Autodesk Fusion 360 part; units mm, degrees
(part 2 of 2)
sketch "Back Honeycomb" plane through (0, 0, 0) normal (0, 0, -1) x (-1, 0, 0)
  line L0 (-88.9, 0) -> (0, 0)
  line L1 (0, 0) -> (0, 22)
  line L2 (0, 22) -> (-88.9, 22)
  line L3 (-88.9, 22) -> (-88.9, 0)
  line L4 (-41.45, 11) -> (-42.95, 13.5981)
  line L5 (-42.95, 13.5981) -> (-45.95, 13.5981)
  line L6 (-45.95, 13.5981) -> (-47.45, 11)
  line L7 (-47.45, 11) -> (-45.95, 8.4019)
  line L8 (-45.95, 8.4019) -> (-42.95, 8.4019)
  line L9 (-42.95, 8.4019) -> (-41.45, 11)
  line L10 (-35.45, 11) -> (-33.95, 8.4019)
  line L11 (-33.95, 8.4019) -> (-30.95, 8.4019)
  line L12 (-30.95, 8.4019) -> (-29.45, 11)
  line L13 (-29.45, 11) -> (-30.95, 13.5981)
  line L14 (-30.95, 13.5981) -> (-33.95, 13.5981)
  line L15 (-33.95, 13.5981) -> (-35.45, 11)
  line L16 (-86.9, 20) -> (-2, 20)
  line L17 (-2, 20) -> (-2, 2)
  line L18 (-2, 2) -> (-86.9, 2)
  line L19 (-86.9, 2) -> (-86.9, 20)
  line L20 (-23.45, 11) -> (-21.95, 8.4019)
  line L21 (-21.95, 8.4019) -> (-18.95, 8.4019)
  line L22 (-18.95, 8.4019) -> (-17.45, 11)
  line L23 (-17.45, 11) -> (-18.95, 13.5981)
  line L24 (-18.95, 13.5981) -> (-21.95, 13.5981)
  line L25 (-21.95, 13.5981) -> (-23.45, 11)
  line L26 (-11.45, 11) -> (-9.95, 8.4019)
  line L27 (-9.95, 8.4019) -> (-6.95, 8.4019)
  line L28 (-6.95, 8.4019) -> (-5.45, 11)
  line L29 (-5.45, 11) -> (-6.95, 13.5981)
  line L30 (-6.95, 13.5981) -> (-9.95, 13.5981)
  line L31 (-9.95, 13.5981) -> (-11.45, 11)
  line L32 (-59.45, 11) -> (-57.95, 8.4019)
  line L33 (-57.95, 8.4019) -> (-54.95, 8.4019)
  line L34 (-54.95, 8.4019) -> (-53.45, 11)
  line L35 (-53.45, 11) -> (-54.95, 13.5981)
  line L36 (-54.95, 13.5981) -> (-57.95, 13.5981)
  line L37 (-57.95, 13.5981) -> (-59.45, 11)
  line L38 (-71.45, 11) -> (-69.95, 8.4019)
  line L39 (-69.95, 8.4019) -> (-66.95, 8.4019)
  line L40 (-66.95, 8.4019) -> (-65.45, 11)
  line L41 (-65.45, 11) -> (-66.95, 13.5981)
  line L42 (-66.95, 13.5981) -> (-69.95, 13.5981)
  line L43 (-69.95, 13.5981) -> (-71.45, 11)
  line L44 (-83.45, 11) -> (-81.95, 8.4019)
  line L45 (-81.95, 8.4019) -> (-78.95, 8.4019)
  line L46 (-78.95, 8.4019) -> (-77.45, 11)
  line L47 (-77.45, 11) -> (-78.95, 13.5981)
  line L48 (-78.95, 13.5981) -> (-81.95, 13.5981)
  line L49 (-81.95, 13.5981) -> (-83.45, 11)
  line L50 (-77.45, 14.5) -> (-75.95, 11.9019)
  line L51 (-75.95, 11.9019) -> (-72.95, 11.9019)
  line L52 (-72.95, 11.9019) -> (-71.45, 14.5)
  line L53 (-71.45, 14.5) -> (-72.95, 17.0981)
  line L54 (-72.95, 17.0981) -> (-75.95, 17.0981)
  line L55 (-75.95, 17.0981) -> (-77.45, 14.5)
  line L56 (-65.45, 14.5) -> (-63.95, 11.9019)
  line L57 (-63.95, 11.9019) -> (-60.95, 11.9019)
  line L58 (-60.95, 11.9019) -> (-59.45, 14.5)
  line L59 (-59.45, 14.5) -> (-60.95, 17.0981)
  line L60 (-60.95, 17.0981) -> (-63.95, 17.0981)
  line L61 (-63.95, 17.0981) -> (-65.45, 14.5)
  line L62 (-53.45, 14.5) -> (-51.95, 11.9019)
  line L63 (-51.95, 11.9019) -> (-48.95, 11.9019)
  line L64 (-48.95, 11.9019) -> (-47.45, 14.5)
  line L65 (-47.45, 14.5) -> (-48.95, 17.0981)
  line L66 (-48.95, 17.0981) -> (-51.95, 17.0981)
  line L67 (-51.95, 17.0981) -> (-53.45, 14.5)
  line L68 (-41.45, 14.5) -> (-39.95, 11.9019)
  line L69 (-39.95, 11.9019) -> (-36.95, 11.9019)
  line L70 (-36.95, 11.9019) -> (-35.45, 14.5)
  line L71 (-35.45, 14.5) -> (-36.95, 17.0981)
  line L72 (-36.95, 17.0981) -> (-39.95, 17.0981)
  line L73 (-39.95, 17.0981) -> (-41.45, 14.5)
  line L74 (-29.45, 14.5) -> (-27.95, 11.9019)
  line L75 (-27.95, 11.9019) -> (-24.95, 11.9019)
  line L76 (-24.95, 11.9019) -> (-23.45, 14.5)
  line L77 (-23.45, 14.5) -> (-24.95, 17.0981)
  line L78 (-24.95, 17.0981) -> (-27.95, 17.0981)
  line L79 (-27.95, 17.0981) -> (-29.45, 14.5)
  line L80 (-17.45, 14.5) -> (-15.95, 11.9019)
  line L81 (-15.95, 11.9019) -> (-12.95, 11.9019)
  line L82 (-12.95, 11.9019) -> (-11.45, 14.5)
  line L83 (-11.45, 14.5) -> (-12.95, 17.0981)
  line L84 (-12.95, 17.0981) -> (-15.95, 17.0981)
  line L85 (-15.95, 17.0981) -> (-17.45, 14.5)
  line L86 (-71.45, 7.5) -> (-72.95, 10.0981)
  line L87 (-72.95, 10.0981) -> (-75.95, 10.0981)
  line L88 (-75.95, 10.0981) -> (-77.45, 7.5)
  line L89 (-77.45, 7.5) -> (-75.95, 4.9019)
  line L90 (-75.95, 4.9019) -> (-72.95, 4.9019)
  line L91 (-72.95, 4.9019) -> (-71.45, 7.5)
  line L92 (-59.45, 7.5) -> (-60.95, 10.0981)
  line L93 (-60.95, 10.0981) -> (-63.95, 10.0981)
  line L94 (-63.95, 10.0981) -> (-65.45, 7.5)
  line L95 (-65.45, 7.5) -> (-63.95, 4.9019)
  line L96 (-60.95, 4.9019) -> (-59.45, 7.5)
  line L97 (-63.95, 4.9019) -> (-60.95, 4.9019)
  line L98 (-47.45, 7.5) -> (-48.95, 10.0981)
  line L99 (-48.95, 10.0981) -> (-51.95, 10.0981)
  line L100 (-51.95, 10.0981) -> (-53.45, 7.5)
  line L101 (-53.45, 7.5) -> (-51.95, 4.9019)
  line L102 (-48.95, 4.9019) -> (-47.45, 7.5)
  line L103 (-51.95, 4.9019) -> (-48.95, 4.9019)
  line L104 (-35.45, 7.5) -> (-36.95, 10.0981)
  line L105 (-36.95, 10.0981) -> (-39.95, 10.0981)
  line L106 (-39.95, 10.0981) -> (-41.45, 7.5)
  line L107 (-41.45, 7.5) -> (-39.95, 4.9019)
  line L108 (-36.95, 4.9019) -> (-35.45, 7.5)
  line L109 (-39.95, 4.9019) -> (-36.95, 4.9019)
  line L110 (-23.45, 7.5) -> (-24.95, 10.0981)
  line L111 (-24.95, 10.0981) -> (-27.95, 10.0981)
  line L112 (-27.95, 10.0981) -> (-29.45, 7.5)
  line L113 (-29.45, 7.5) -> (-27.95, 4.9019)
  line L114 (-24.95, 4.9019) -> (-23.45, 7.5)
  line L115 (-27.95, 4.9019) -> (-24.95, 4.9019)
  line L116 (-11.45, 7.5) -> (-12.95, 10.0981)
  line L117 (-12.95, 10.0981) -> (-15.95, 10.0981)
  line L118 (-15.95, 10.0981) -> (-17.45, 7.5)
  line L119 (-17.45, 7.5) -> (-15.95, 4.9019)
  line L120 (-12.95, 4.9019) -> (-11.45, 7.5)
  line L121 (-15.95, 4.9019) -> (-12.95, 4.9019)
  line L122 (-83.45, 18) -> (-81.95, 15.4019)
  line L123 (-81.95, 15.4019) -> (-78.95, 15.4019)
  line L124 (-78.95, 15.4019) -> (-77.45, 18)
  line L125 (-77.45, 18) -> (-78.95, 20.5981)
  line L126 (-78.95, 20.5981) -> (-81.95, 20.5981)
  line L127 (-81.95, 20.5981) -> (-83.45, 18)
  line L128 (-71.45, 18) -> (-69.95, 15.4019)
  line L129 (-69.95, 15.4019) -> (-66.95, 15.4019)
  line L130 (-66.95, 15.4019) -> (-65.45, 18)
  line L131 (-65.45, 18) -> (-66.95, 20.5981)
  line L132 (-69.95, 20.5981) -> (-71.45, 18)
  line L133 (-66.95, 20.5981) -> (-69.95, 20.5981)
  line L134 (-59.45, 18) -> (-57.95, 15.4019)
  line L135 (-57.95, 15.4019) -> (-54.95, 15.4019)
  line L136 (-54.95, 15.4019) -> (-53.45, 18)
  line L137 (-53.45, 18) -> (-54.95, 20.5981)
  line L138 (-57.95, 20.5981) -> (-59.45, 18)
  line L139 (-54.95, 20.5981) -> (-57.95, 20.5981)
  line L140 (-47.45, 18) -> (-45.95, 15.4019)
  line L141 (-45.95, 15.4019) -> (-42.95, 15.4019)
  line L142 (-42.95, 15.4019) -> (-41.45, 18)
  line L143 (-41.45, 18) -> (-42.95, 20.5981)
  line L144 (-45.95, 20.5981) -> (-47.45, 18)
  line L145 (-42.95, 20.5981) -> (-45.95, 20.5981)
  line L146 (-35.45, 18) -> (-33.95, 15.4019)
  line L147 (-33.95, 15.4019) -> (-30.95, 15.4019)
  line L148 (-30.95, 15.4019) -> (-29.45, 18)
  line L149 (-29.45, 18) -> (-30.95, 20.5981)
  line L150 (-33.95, 20.5981) -> (-35.45, 18)
  line L151 (-30.95, 20.5981) -> (-33.95, 20.5981)
  line L152 (-23.45, 18) -> (-21.95, 15.4019)
  line L153 (-21.95, 15.4019) -> (-18.95, 15.4019)
  line L154 (-18.95, 15.4019) -> (-17.45, 18)
  line L155 (-17.45, 18) -> (-18.95, 20.5981)
  line L156 (-21.95, 20.5981) -> (-23.45, 18)
  line L157 (-18.95, 20.5981) -> (-21.95, 20.5981)
  line L158 (-11.45, 18) -> (-9.95, 15.4019)
  line L159 (-9.95, 15.4019) -> (-6.95, 15.4019)
  line L160 (-6.95, 15.4019) -> (-5.45, 18)
  line L161 (-5.45, 18) -> (-6.95, 20.5981)
  line L162 (-9.95, 20.5981) -> (-11.45, 18)
  line L163 (-6.95, 20.5981) -> (-9.95, 20.5981)
  line L164 (-83.45, 4) -> (-81.95, 1.4019)
  line L165 (-81.95, 1.4019) -> (-78.95, 1.4019)
  line L166 (-78.95, 1.4019) -> (-77.45, 4)
  line L167 (-77.45, 4) -> (-78.95, 6.5981)
  line L168 (-78.95, 6.5981) -> (-81.95, 6.5981)
  line L169 (-81.95, 6.5981) -> (-83.45, 4)
  line L170 (-71.45, 4) -> (-69.95, 1.4019)
  line L171 (-69.95, 1.4019) -> (-66.95, 1.4019)
  line L172 (-66.95, 1.4019) -> (-65.45, 4)
  line L173 (-65.45, 4) -> (-66.95, 6.5981)
  line L174 (-69.95, 6.5981) -> (-71.45, 4)
  line L175 (-66.95, 6.5981) -> (-69.95, 6.5981)
  line L176 (-59.45, 4) -> (-57.95, 1.4019)
  line L177 (-57.95, 1.4019) -> (-54.95, 1.4019)
  line L178 (-54.95, 1.4019) -> (-53.45, 4)
  line L179 (-53.45, 4) -> (-54.95, 6.5981)
  line L180 (-57.95, 6.5981) -> (-59.45, 4)
  line L181 (-54.95, 6.5981) -> (-57.95, 6.5981)
  line L182 (-47.45, 4) -> (-45.95, 1.4019)
  line L183 (-45.95, 1.4019) -> (-42.95, 1.4019)
  line L184 (-42.95, 1.4019) -> (-41.45, 4)
  line L185 (-41.45, 4) -> (-42.95, 6.5981)
  line L186 (-45.95, 6.5981) -> (-47.45, 4)
  line L187 (-42.95, 6.5981) -> (-45.95, 6.5981)
  line L188 (-35.45, 4) -> (-33.95, 1.4019)
  line L189 (-33.95, 1.4019) -> (-30.95, 1.4019)
  line L190 (-30.95, 1.4019) -> (-29.45, 4)
  line L191 (-29.45, 4) -> (-30.95, 6.5981)
  line L192 (-33.95, 6.5981) -> (-35.45, 4)
  line L193 (-30.95, 6.5981) -> (-33.95, 6.5981)
  line L194 (-23.45, 4) -> (-21.95, 1.4019)
  line L195 (-21.95, 1.4019) -> (-18.95, 1.4019)
  line L196 (-18.95, 1.4019) -> (-17.45, 4)
  line L197 (-17.45, 4) -> (-18.95, 6.5981)
  line L198 (-21.95, 6.5981) -> (-23.45, 4)
  line L199 (-18.95, 6.5981) -> (-21.95, 6.5981)
  line L200 (-11.45, 4) -> (-9.95, 1.4019)
  line L201 (-9.95, 1.4019) -> (-6.95, 1.4019)
  line L202 (-6.95, 1.4019) -> (-5.45, 4)
  line L203 (-5.45, 4) -> (-6.95, 6.5981)
  line L204 (-9.95, 6.5981) -> (-11.45, 4)
  line L205 (-6.95, 6.5981) -> (-9.95, 6.5981)
  line L206 (0.55, 14.5) -> (-0.95, 17.0981)
  line L207 (-0.95, 17.0981) -> (-3.95, 17.0981)
  line L208 (-3.95, 17.0981) -> (-5.45, 14.5)
  line L209 (-5.45, 14.5) -> (-3.95, 11.9019)
  line L210 (-3.95, 11.9019) -> (-0.95, 11.9019)
  line L211 (-0.95, 11.9019) -> (0.55, 14.5)
  line L212 (-5.45, 7.5) -> (-3.95, 4.9019)
  line L213 (-3.95, 4.9019) -> (-0.95, 4.9019)
  line L214 (-0.95, 4.9019) -> (0.55, 7.5)
  line L215 (0.55, 7.5) -> (-0.95, 10.0981)
  line L216 (-3.95, 10.0981) -> (-5.45, 7.5)
  line L217 (-0.95, 10.0981) -> (-3.95, 10.0981)
  line L218 (-89.45, 14.5) -> (-87.95, 11.9019)
  line L219 (-87.95, 11.9019) -> (-84.95, 11.9019)
  line L220 (-84.95, 11.9019) -> (-83.45, 14.5)
  line L221 (-83.45, 14.5) -> (-84.95, 17.0981)
  line L222 (-84.95, 17.0981) -> (-87.95, 17.0981)
  line L223 (-87.95, 17.0981) -> (-89.45, 14.5)
  line L224 (-89.45, 7.5) -> (-87.95, 4.9019)
  line L225 (-87.95, 4.9019) -> (-84.95, 4.9019)
  line L226 (-84.95, 4.9019) -> (-83.45, 7.5)
  line L227 (-83.45, 7.5) -> (-84.95, 10.0981)
  line L228 (-87.95, 10.0981) -> (-89.45, 7.5)
  line L229 (-84.95, 10.0981) -> (-87.95, 10.0981)
  line L230 (-77.45, 21.5) -> (-75.95, 18.9019)
  line L231 (-75.95, 18.9019) -> (-72.95, 18.9019)
  line L232 (-72.95, 18.9019) -> (-71.45, 21.5)
  line L233 (-71.45, 21.5) -> (-72.95, 24.0981)
  line L234 (-72.95, 24.0981) -> (-75.95, 24.0981)
  line L235 (-75.95, 24.0981) -> (-77.45, 21.5)
  line L236 (-65.45, 21.5) -> (-63.95, 18.9019)
  line L237 (-63.95, 18.9019) -> (-60.95, 18.9019)
  line L238 (-60.95, 18.9019) -> (-59.45, 21.5)
  line L239 (-59.45, 21.5) -> (-60.95, 24.0981)
  line L240 (-63.95, 24.0981) -> (-65.45, 21.5)
  line L241 (-60.95, 24.0981) -> (-63.95, 24.0981)
  line L242 (-53.45, 21.5) -> (-51.95, 18.9019)
  line L243 (-51.95, 18.9019) -> (-48.95, 18.9019)
  line L244 (-48.95, 18.9019) -> (-47.45, 21.5)
  line L245 (-47.45, 21.5) -> (-48.95, 24.0981)
  line L246 (-51.95, 24.0981) -> (-53.45, 21.5)
  line L247 (-48.95, 24.0981) -> (-51.95, 24.0981)
  line L248 (-41.45, 21.5) -> (-39.95, 18.9019)
  line L249 (-39.95, 18.9019) -> (-36.95, 18.9019)
  line L250 (-36.95, 18.9019) -> (-35.45, 21.5)
  line L251 (-35.45, 21.5) -> (-36.95, 24.0981)
  line L252 (-39.95, 24.0981) -> (-41.45, 21.5)
  line L253 (-36.95, 24.0981) -> (-39.95, 24.0981)
  line L254 (-29.45, 21.5) -> (-27.95, 18.9019)
  line L255 (-27.95, 18.9019) -> (-24.95, 18.9019)
  line L256 (-24.95, 18.9019) -> (-23.45, 21.5)
  line L257 (-23.45, 21.5) -> (-24.95, 24.0981)
  line L258 (-27.95, 24.0981) -> (-29.45, 21.5)
  line L259 (-24.95, 24.0981) -> (-27.95, 24.0981)
  line L260 (-17.45, 21.5) -> (-15.95, 18.9019)
  line L261 (-15.95, 18.9019) -> (-12.95, 18.9019)
  line L262 (-12.95, 18.9019) -> (-11.45, 21.5)
  line L263 (-11.45, 21.5) -> (-12.95, 24.0981)
  line L264 (-15.95, 24.0981) -> (-17.45, 21.5)
  line L265 (-12.95, 24.0981) -> (-15.95, 24.0981)
  line L266 (-5.45, 21.5) -> (-3.95, 18.9019)
  line L267 (-3.95, 18.9019) -> (-0.95, 18.9019)
  line L268 (-0.95, 18.9019) -> (0.55, 21.5)
  line L269 (0.55, 21.5) -> (-0.95, 24.0981)
  line L270 (-3.95, 24.0981) -> (-5.45, 21.5)
  line L271 (-0.95, 24.0981) -> (-3.95, 24.0981)
  line L272 (-77.45, 0.5) -> (-75.95, -2.0981)
  line L273 (-75.95, -2.0981) -> (-72.95, -2.0981)
  line L274 (-72.95, -2.0981) -> (-71.45, 0.5)
  line L275 (-71.45, 0.5) -> (-72.95, 3.0981)
  line L276 (-72.95, 3.0981) -> (-75.95, 3.0981)
  line L277 (-75.95, 3.0981) -> (-77.45, 0.5)
  line L278 (-65.45, 0.5) -> (-63.95, -2.0981)
  line L279 (-63.95, -2.0981) -> (-60.95, -2.0981)
  line L280 (-60.95, -2.0981) -> (-59.45, 0.5)
  line L281 (-59.45, 0.5) -> (-60.95, 3.0981)
  line L282 (-63.95, 3.0981) -> (-65.45, 0.5)
  line L283 (-60.95, 3.0981) -> (-63.95, 3.0981)
  line L284 (-53.45, 0.5) -> (-51.95, -2.0981)
  line L285 (-51.95, -2.0981) -> (-48.95, -2.0981)
  line L286 (-48.95, -2.0981) -> (-47.45, 0.5)
  line L287 (-47.45, 0.5) -> (-48.95, 3.0981)
  line L288 (-51.95, 3.0981) -> (-53.45, 0.5)
  line L289 (-48.95, 3.0981) -> (-51.95, 3.0981)
  line L290 (-41.45, 0.5) -> (-39.95, -2.0981)
  line L291 (-39.95, -2.0981) -> (-36.95, -2.0981)
  line L292 (-36.95, -2.0981) -> (-35.45, 0.5)
  line L293 (-35.45, 0.5) -> (-36.95, 3.0981)
  line L294 (-39.95, 3.0981) -> (-41.45, 0.5)
  line L295 (-36.95, 3.0981) -> (-39.95, 3.0981)
  line L296 (-29.45, 0.5) -> (-27.95, -2.0981)
  line L297 (-27.95, -2.0981) -> (-24.95, -2.0981)
  line L298 (-24.95, -2.0981) -> (-23.45, 0.5)
  line L299 (-23.45, 0.5) -> (-24.95, 3.0981)
  line L300 (-27.95, 3.0981) -> (-29.45, 0.5)
  line L301 (-24.95, 3.0981) -> (-27.95, 3.0981)
  line L302 (-17.45, 0.5) -> (-15.95, -2.0981)
  line L303 (-15.95, -2.0981) -> (-12.95, -2.0981)
  line L304 (-12.95, -2.0981) -> (-11.45, 0.5)
  line L305 (-11.45, 0.5) -> (-12.95, 3.0981)
  line L306 (-15.95, 3.0981) -> (-17.45, 0.5)
  line L307 (-12.95, 3.0981) -> (-15.95, 3.0981)
  line L308 (-5.45, 0.5) -> (-3.95, -2.0981)
  line L309 (-3.95, -2.0981) -> (-0.95, -2.0981)
  line L310 (-0.95, -2.0981) -> (0.55, 0.5)
  line L311 (0.55, 0.5) -> (-0.95, 3.0981)
  line L312 (-3.95, 3.0981) -> (-5.45, 0.5)
  line L313 (-0.95, 3.0981) -> (-3.95, 3.0981)
  line L314 (-89.45, 21.5) -> (-87.95, 18.9019)
  line L315 (-87.95, 18.9019) -> (-84.95, 18.9019)
  line L316 (-84.95, 18.9019) -> (-83.45, 21.5)
  line L317 (-83.45, 21.5) -> (-84.95, 24.0981)
  line L318 (-84.95, 24.0981) -> (-87.95, 24.0981)
  line L319 (-87.95, 24.0981) -> (-89.45, 21.5)
  line L320 (-83.45, 0.5) -> (-84.95, 3.0981)
  line L321 (-84.95, 3.0981) -> (-87.95, 3.0981)
  line L322 (-87.95, 3.0981) -> (-89.45, 0.5)
  line L323 (-89.45, 0.5) -> (-87.95, -2.0981)
  line L324 (-87.95, -2.0981) -> (-84.95, -2.0981)
  line L325 (-84.95, -2.0981) -> (-83.45, 0.5)
  line L326 (-8.45, 20.5981) -> (-8.45, 15.4019) construction
  line L327 (-32.45, 20.5981) -> (-32.45, 15.4019) construction
  line L328 (-44.45, 20.5981) -> (-44.45, 15.4019) construction
  line L329 (-80.45, 20.5981) -> (-80.45, 15.4019) construction
  line L330 (-88.9, 18.0734) -> (0, 18) construction
  point P0 (-44.45, 11)
  point P1 (-44.45, 11)
  point P2 (-44.45, 11)
  point P3 (-2, 2)
  dimension "d240" = 5.1962
  dimension "d241" = 5.45
  dimension "d242" = 88.9
  measures "d240" distance of L326.start L326.end
  measures "d241" distance of L160.end L330.end
  measures "d242" distance of L330.end L330.start
extrude "Extrude11" cut sketch "Back Honeycomb" against normal blind 2 contours L18 L19 L320 L321 | L18 L275 L276 L277 | L18 L164 L166 L167 L168 L169 | L19 L225 L226 L227 L229 | L18 L281 L282 L283 | L18 L170 L172 L173 L174 L175 | L19 L219 L220 L221 L222 | L18 L287 L288 L289 | L18 L176 L178 L179 L180 L181 | L16 L19 L315 L316 | L18 L293 L294 L295 | L18 L182 L184 L185 L186 L187 | L16 L230 L231 L232 | L16 L122 L123 L124 L125 L127 | L18 L299 L300 L301 | L18 L188 L190 L191 L192 L193 | L16 L236 L237 L238 | L16 L128 L129 L130 L131 L132 | L18 L305 L306 L307 | L18 L194 L196 L197 L198 L199 | L16 L242 L243 L244 | L16 L134 L135 L136 L137 L138 | L17 L18 L312 L313 | L18 L200 L202 L203 L204 L205 | L16 L248 L249 L250 | L16 L140 L141 L142 L143 L144 | L17 L212 L213 L216 L217 | L16 L254 L255 L256 | L16 L146 L147 L148 L149 L150 | L17 L207 L208 L209 L210 | L16 L260 L261 L262 | L16 L152 L153 L154 L155 L156 | L16 L17 L266 L267 | L16 L158 L159 L160 L161 L162 | L4 L5 L6 L7 L8 L9 | L10 L11 L12 L13 L14 L15 | L20 L21 L22 L23 L24 L25 | L26 L27 L28 L29 L30 L31 | L32 L33 L34 L35 L36 L37 | L38 L39 L40 L41 L42 L43 | L44 L45 L46 L47 L48 L49 | L50 L51 L52 L53 L54 L55 | L56 L57 L58 L59 L60 L61 | L62 L63 L64 L65 L66 L67 | L68 L69 L70 L71 L72 L73 | L74 L75 L76 L77 L78 L79 | L80 L81 L82 L83 L84 L85 | L86 L87 L88 L89 L90 L91 | L92 L93 L94 L95 L96 L97 | L98 L99 L100 L101 L102 L103 | L104 L105 L106 L107 L108 L109 | L110 L111 L112 L113 L114 L115 | L116 L117 L118 L119 L120 L121 bodies 2
extrude "Extrude12" cut sketch "Bottom Honeycomb" along normal blind 2 contours L493 L513 L514 L515 L517 | L485 L486 L487 L492 A2 | L493 L507 L508 L509 L511 | L492 L493 A2 L556 | L493 L500 L501 L504 L505 | L422 L423 L424 L425 L427 L492 | L476 L477 L478 L492 | L428 L429 L430 L431 A1 | L392 L393 L394 L395 L396 L492 | L470 L471 L472 L492 | L362 L363 L364 L365 L367 L490 | L386 L387 L388 L389 L390 L490 | L398 L399 L400 L401 L402 L492 | L368 L369 L372 L490 A8 | L491 L524 L529 | L442 L443 L444 L445 A0 | L380 L381 L382 L383 L384 L490 | L369 L370 L371 L490 A8 | L464 L465 L466 L492 | L491 L530 L534 | L374 L375 L376 L377 L378 L490 | L404 L405 L406 L407 L408 L492 | L491 L536 L540 | L458 L459 L460 L492 | L446 L449 L450 L451 A3 | L410 L411 L412 L413 L414 L492 | L491 A3 L542 | L452 L453 L454 L492 | L492 A3 L497 L498 L499 | L416 L417 L418 L419 L420 L492 bodies 1
sketch "Non-USB Honeycomb" plane through (88.9, 0, 0) normal (1, 0, 0) x (0, 0, -1)
  line L0 (-47.6, 0) -> (0, 0)
  line L1 (0, 0) -> (0, 22)
  line L2 (0, 22) -> (-47.6, 22)
  line L3 (-47.6, 22) -> (-47.6, 0)
  line L4 (-45.6, 20) -> (-2, 20)
  line L5 (-2, 20) -> (-2, 2)
  line L6 (-2, 2) -> (-45.6, 2)
  line L7 (-45.6, 2) -> (-45.6, 20)
  line L8 (-45.6, 11) -> (-2, 11) construction
  line L9 (-23.8, 20) -> (-23.8, 2) construction
  line L10 (-20.8, 11) -> (-22.3, 13.5981)
  line L11 (-22.3, 13.5981) -> (-25.3, 13.5981)
  line L12 (-25.3, 13.5981) -> (-26.8, 11)
  line L13 (-26.8, 11) -> (-25.3, 8.4019)
  line L14 (-25.3, 8.4019) -> (-22.3, 8.4019)
  line L15 (-22.3, 8.4019) -> (-20.8, 11)
  line L16 (-14.8, 11) -> (-13.3, 8.4019)
  line L17 (-13.3, 8.4019) -> (-10.3, 8.4019)
  line L18 (-10.3, 8.4019) -> (-8.8, 11)
  line L19 (-8.8, 11) -> (-10.3, 13.5981)
  line L20 (-10.3, 13.5981) -> (-13.3, 13.5981)
  line L21 (-13.3, 13.5981) -> (-14.8, 11)
  line L22 (-2.8, 11) -> (-1.3, 8.4019)
  line L23 (-1.3, 8.4019) -> (1.7, 8.4019)
  line L24 (1.7, 8.4019) -> (3.2, 11)
  line L25 (3.2, 11) -> (1.7, 13.5981)
  line L26 (1.7, 13.5981) -> (-1.3, 13.5981)
  line L27 (-1.3, 13.5981) -> (-2.8, 11)
  line L28 (-38.8, 11) -> (-37.3, 8.4019)
  line L29 (-37.3, 8.4019) -> (-34.3, 8.4019)
  line L30 (-34.3, 8.4019) -> (-32.8, 11)
  line L31 (-32.8, 11) -> (-34.3, 13.5981)
  line L32 (-34.3, 13.5981) -> (-37.3, 13.5981)
  line L33 (-37.3, 13.5981) -> (-38.8, 11)
  line L34 (-50.8, 11) -> (-49.3, 8.4019)
  line L35 (-49.3, 8.4019) -> (-46.3, 8.4019)
  line L36 (-46.3, 8.4019) -> (-44.8, 11)
  line L37 (-44.8, 11) -> (-46.3, 13.5981)
  line L38 (-46.3, 13.5981) -> (-49.3, 13.5981)
  line L39 (-49.3, 13.5981) -> (-50.8, 11)
  line L40 (-50.8, 18) -> (-49.3, 15.4019)
  line L41 (-49.3, 15.4019) -> (-46.3, 15.4019)
  line L42 (-46.3, 15.4019) -> (-44.8, 18)
  line L43 (-44.8, 18) -> (-46.3, 20.5981)
  line L44 (-46.3, 20.5981) -> (-49.3, 20.5981)
  line L45 (-49.3, 20.5981) -> (-50.8, 18)
  line L46 (-38.8, 18) -> (-37.3, 15.4019)
  line L47 (-37.3, 15.4019) -> (-34.3, 15.4019)
  line L48 (-34.3, 15.4019) -> (-32.8, 18)
  line L49 (-32.8, 18) -> (-34.3, 20.5981)
  line L50 (-37.3, 20.5981) -> (-38.8, 18)
  line L51 (-34.3, 20.5981) -> (-37.3, 20.5981)
  line L52 (-26.8, 18) -> (-25.3, 15.4019)
  line L53 (-25.3, 15.4019) -> (-22.3, 15.4019)
  line L54 (-22.3, 15.4019) -> (-20.8, 18)
  line L55 (-20.8, 18) -> (-22.3, 20.5981)
  line L56 (-25.3, 20.5981) -> (-26.8, 18)
  line L57 (-22.3, 20.5981) -> (-25.3, 20.5981)
  line L58 (-14.8, 18) -> (-13.3, 15.4019)
  line L59 (-13.3, 15.4019) -> (-10.3, 15.4019)
  line L60 (-10.3, 15.4019) -> (-8.8, 18)
  line L61 (-8.8, 18) -> (-10.3, 20.5981)
  line L62 (-13.3, 20.5981) -> (-14.8, 18)
  line L63 (-10.3, 20.5981) -> (-13.3, 20.5981)
  line L64 (-2.8, 18) -> (-1.3, 15.4019)
  line L65 (-1.3, 15.4019) -> (1.7, 15.4019)
  line L66 (1.7, 15.4019) -> (3.2, 18)
  line L67 (3.2, 18) -> (1.7, 20.5981)
  line L68 (-1.3, 20.5981) -> (-2.8, 18)
  line L69 (1.7, 20.5981) -> (-1.3, 20.5981)
  line L70 (-50.8, 4) -> (-49.3, 1.4019)
  line L71 (-49.3, 1.4019) -> (-46.3, 1.4019)
  line L72 (-46.3, 1.4019) -> (-44.8, 4)
  line L73 (-44.8, 4) -> (-46.3, 6.5981)
  line L74 (-46.3, 6.5981) -> (-49.3, 6.5981)
  line L75 (-49.3, 6.5981) -> (-50.8, 4)
  line L76 (-38.8, 4) -> (-37.3, 1.4019)
  line L77 (-37.3, 1.4019) -> (-34.3, 1.4019)
  line L78 (-34.3, 1.4019) -> (-32.8, 4)
  line L79 (-32.8, 4) -> (-34.3, 6.5981)
  line L80 (-37.3, 6.5981) -> (-38.8, 4)
  line L81 (-34.3, 6.5981) -> (-37.3, 6.5981)
  line L82 (-26.8, 4) -> (-25.3, 1.4019)
  line L83 (-25.3, 1.4019) -> (-22.3, 1.4019)
  line L84 (-22.3, 1.4019) -> (-20.8, 4)
  line L85 (-20.8, 4) -> (-22.3, 6.5981)
  line L86 (-25.3, 6.5981) -> (-26.8, 4)
  line L87 (-22.3, 6.5981) -> (-25.3, 6.5981)
  line L88 (-14.8, 4) -> (-13.3, 1.4019)
  line L89 (-13.3, 1.4019) -> (-10.3, 1.4019)
  line L90 (-10.3, 1.4019) -> (-8.8, 4)
  line L91 (-8.8, 4) -> (-10.3, 6.5981)
  line L92 (-13.3, 6.5981) -> (-14.8, 4)
  line L93 (-10.3, 6.5981) -> (-13.3, 6.5981)
  line L94 (-2.8, 4) -> (-1.3, 1.4019)
  line L95 (-1.3, 1.4019) -> (1.7, 1.4019)
  line L96 (1.7, 1.4019) -> (3.2, 4)
  line L97 (3.2, 4) -> (1.7, 6.5981)
  line L98 (-1.3, 6.5981) -> (-2.8, 4)
  line L99 (1.7, 6.5981) -> (-1.3, 6.5981)
  line L100 (-32.8, 14.5) -> (-31.3, 11.9019)
  line L101 (-31.3, 11.9019) -> (-28.3, 11.9019)
  line L102 (-28.3, 11.9019) -> (-26.8, 14.5)
  line L103 (-26.8, 14.5) -> (-28.3, 17.0981)
  line L104 (-28.3, 17.0981) -> (-31.3, 17.0981)
  line L105 (-31.3, 17.0981) -> (-32.8, 14.5)
  line L106 (-20.8, 14.5) -> (-19.3, 11.9019)
  line L107 (-19.3, 11.9019) -> (-16.3, 11.9019)
  line L108 (-16.3, 11.9019) -> (-14.8, 14.5)
  line L109 (-14.8, 14.5) -> (-16.3, 17.0981)
  line L110 (-16.3, 17.0981) -> (-19.3, 17.0981)
  line L111 (-19.3, 17.0981) -> (-20.8, 14.5)
  line L112 (-8.8, 14.5) -> (-7.3, 11.9019)
  line L113 (-7.3, 11.9019) -> (-4.3, 11.9019)
  line L114 (-4.3, 11.9019) -> (-2.8, 14.5)
  line L115 (-2.8, 14.5) -> (-4.3, 17.0981)
  line L116 (-4.3, 17.0981) -> (-7.3, 17.0981)
  line L117 (-7.3, 17.0981) -> (-8.8, 14.5)
  line L118 (-44.8, 14.5) -> (-43.3, 11.9019)
  line L119 (-43.3, 11.9019) -> (-40.3, 11.9019)
  line L120 (-40.3, 11.9019) -> (-38.8, 14.5)
  line L121 (-38.8, 14.5) -> (-40.3, 17.0981)
  line L122 (-40.3, 17.0981) -> (-43.3, 17.0981)
  line L123 (-43.3, 17.0981) -> (-44.8, 14.5)
  line L124 (-44.8, 21.5) -> (-43.3, 18.9019)
  line L125 (-43.3, 18.9019) -> (-40.3, 18.9019)
  line L126 (-40.3, 18.9019) -> (-38.8, 21.5)
  line L127 (-38.8, 21.5) -> (-40.3, 24.0981)
  line L128 (-40.3, 24.0981) -> (-43.3, 24.0981)
  line L129 (-43.3, 24.0981) -> (-44.8, 21.5)
  line L130 (-32.8, 21.5) -> (-31.3, 18.9019)
  line L131 (-31.3, 18.9019) -> (-28.3, 18.9019)
  line L132 (-28.3, 18.9019) -> (-26.8, 21.5)
  line L133 (-26.8, 21.5) -> (-28.3, 24.0981)
  line L134 (-31.3, 24.0981) -> (-32.8, 21.5)
  line L135 (-28.3, 24.0981) -> (-31.3, 24.0981)
  line L136 (-20.8, 21.5) -> (-19.3, 18.9019)
  line L137 (-19.3, 18.9019) -> (-16.3, 18.9019)
  line L138 (-16.3, 18.9019) -> (-14.8, 21.5)
  line L139 (-14.8, 21.5) -> (-16.3, 24.0981)
  line L140 (-19.3, 24.0981) -> (-20.8, 21.5)
  line L141 (-16.3, 24.0981) -> (-19.3, 24.0981)
  line L142 (-8.8, 21.5) -> (-7.3, 18.9019)
  line L143 (-7.3, 18.9019) -> (-4.3, 18.9019)
  line L144 (-4.3, 18.9019) -> (-2.8, 21.5)
  line L145 (-2.8, 21.5) -> (-4.3, 24.0981)
  line L146 (-7.3, 24.0981) -> (-8.8, 21.5)
  line L147 (-4.3, 24.0981) -> (-7.3, 24.0981)
  line L148 (-44.8, 7.5) -> (-43.3, 4.9019)
  line L149 (-43.3, 4.9019) -> (-40.3, 4.9019)
  line L150 (-40.3, 4.9019) -> (-38.8, 7.5)
  line L151 (-38.8, 7.5) -> (-40.3, 10.0981)
  line L152 (-40.3, 10.0981) -> (-43.3, 10.0981)
  line L153 (-43.3, 10.0981) -> (-44.8, 7.5)
  line L154 (-32.8, 7.5) -> (-31.3, 4.9019)
  line L155 (-31.3, 4.9019) -> (-28.3, 4.9019)
  line L156 (-28.3, 4.9019) -> (-26.8, 7.5)
  line L157 (-26.8, 7.5) -> (-28.3, 10.0981)
  line L158 (-31.3, 10.0981) -> (-32.8, 7.5)
  line L159 (-28.3, 10.0981) -> (-31.3, 10.0981)
  line L160 (-20.8, 7.5) -> (-19.3, 4.9019)
  line L161 (-19.3, 4.9019) -> (-16.3, 4.9019)
  line L162 (-16.3, 4.9019) -> (-14.8, 7.5)
  line L163 (-14.8, 7.5) -> (-16.3, 10.0981)
  line L164 (-19.3, 10.0981) -> (-20.8, 7.5)
  line L165 (-16.3, 10.0981) -> (-19.3, 10.0981)
  line L166 (-8.8, 7.5) -> (-7.3, 4.9019)
  line L167 (-7.3, 4.9019) -> (-4.3, 4.9019)
  line L168 (-4.3, 4.9019) -> (-2.8, 7.5)
  line L169 (-2.8, 7.5) -> (-4.3, 10.0981)
  line L170 (-7.3, 10.0981) -> (-8.8, 7.5)
  line L171 (-4.3, 10.0981) -> (-7.3, 10.0981)
  line L172 (-44.8, 0.5) -> (-43.3, -2.0981)
  line L173 (-43.3, -2.0981) -> (-40.3, -2.0981)
  line L174 (-40.3, -2.0981) -> (-38.8, 0.5)
  line L175 (-38.8, 0.5) -> (-40.3, 3.0981)
  line L176 (-40.3, 3.0981) -> (-43.3, 3.0981)
  line L177 (-43.3, 3.0981) -> (-44.8, 0.5)
  line L178 (-32.8, 0.5) -> (-31.3, -2.0981)
  line L179 (-31.3, -2.0981) -> (-28.3, -2.0981)
  line L180 (-28.3, -2.0981) -> (-26.8, 0.5)
  line L181 (-26.8, 0.5) -> (-28.3, 3.0981)
  line L182 (-31.3, 3.0981) -> (-32.8, 0.5)
  line L183 (-28.3, 3.0981) -> (-31.3, 3.0981)
  line L184 (-20.8, 0.5) -> (-19.3, -2.0981)
  line L185 (-19.3, -2.0981) -> (-16.3, -2.0981)
  line L186 (-16.3, -2.0981) -> (-14.8, 0.5)
  line L187 (-14.8, 0.5) -> (-16.3, 3.0981)
  line L188 (-19.3, 3.0981) -> (-20.8, 0.5)
  line L189 (-16.3, 3.0981) -> (-19.3, 3.0981)
  line L190 (-8.8, 0.5) -> (-7.3, -2.0981)
  line L191 (-7.3, -2.0981) -> (-4.3, -2.0981)
  line L192 (-4.3, -2.0981) -> (-2.8, 0.5)
  line L193 (-2.8, 0.5) -> (-4.3, 3.0981)
  line L194 (-7.3, 3.0981) -> (-8.8, 0.5)
  line L195 (-4.3, 3.0981) -> (-7.3, 3.0981)
  point P0 (-2, 2)
  point P1 (-2, 11)
  point P2 (-23.8, 11)
extrude "Extrude13" cut sketch "Non-USB Honeycomb" against normal blind 2 contours L6 L175 L176 L177 | L7 L72 L73 | L6 L181 L182 L183 | L6 L76 L78 L79 L80 L81 | L7 L36 L37 | L6 L187 L188 L189 | L6 L82 L84 L85 L86 L87 | L7 L42 L43 | L6 L193 L194 L195 | L6 L88 L90 L91 L92 L93 | L4 L124 L125 L126 | L5 L94 L98 | L4 L130 L131 L132 | L4 L46 L47 L48 L49 L50 | L5 L22 L27 | L4 L136 L137 L138 | L4 L52 L53 L54 L55 L56 | L5 L64 L68 | L4 L142 L143 L144 | L4 L58 L59 L60 L61 L62 | L10 L11 L12 L13 L14 L15 | L16 L17 L18 L19 L20 L21 | L28 L29 L30 L31 L32 L33 | L100 L101 L102 L103 L104 L105 | L106 L107 L108 L109 L110 L111 | L112 L113 L114 L115 L116 L117 | L118 L119 L120 L121 L122 L123 | L148 L149 L150 L151 L152 L153 | L154 L155 L156 L157 L158 L159 | L160 L161 L162 L163 L164 L165 | L166 L167 L168 L169 L170 L171 bodies 2
sketch "USB Honeycomb" plane through (0, 0, 0) normal (-1, 0, 0) x (0, 0, 1)
  line L0 (14.33, 10) -> (30.93, 10)
  line L1 (30.93, 10) -> (30.93, 3)
  line L2 (30.93, 3) -> (14.33, 3)
  line L3 (14.33, 3) -> (14.33, 10)
  line L4 (0, 0) -> (47.6, 0)
  line L5 (47.6, 0) -> (47.6, 22)
  line L6 (47.6, 22) -> (0, 22)
  line L7 (0, 22) -> (0, 0)
  line L8 (2, 20) -> (45.6, 20)
  line L9 (45.6, 20) -> (45.6, 2)
  line L10 (45.6, 2) -> (2, 2)
  line L11 (2, 2) -> (2, 20)
  line L12 (26.8, 11) -> (25.3, 13.5981)
  line L13 (25.3, 13.5981) -> (22.3, 13.5981)
  line L14 (22.3, 13.5981) -> (20.8, 11)
  line L15 (20.8, 11) -> (22.3, 8.4019)
  line L16 (22.3, 8.4019) -> (25.3, 8.4019)
  line L17 (25.3, 8.4019) -> (26.8, 11)
  line L18 (32.8, 11) -> (34.3, 8.4019)
  line L19 (34.3, 8.4019) -> (37.3, 8.4019)
  line L20 (37.3, 8.4019) -> (38.8, 11)
  line L21 (38.8, 11) -> (37.3, 13.5981)
  line L22 (37.3, 13.5981) -> (34.3, 13.5981)
  line L23 (34.3, 13.5981) -> (32.8, 11)
  line L24 (44.8, 11) -> (46.3, 8.4019)
  line L25 (46.3, 8.4019) -> (49.3, 8.4019)
  line L26 (49.3, 8.4019) -> (50.8, 11)
  line L27 (50.8, 11) -> (49.3, 13.5981)
  line L28 (49.3, 13.5981) -> (46.3, 13.5981)
  line L29 (46.3, 13.5981) -> (44.8, 11)
  line L30 (8.8, 11) -> (10.3, 8.4019)
  line L31 (10.3, 8.4019) -> (13.3, 8.4019)
  line L32 (13.3, 8.4019) -> (14.8, 11)
  line L33 (14.8, 11) -> (13.3, 13.5981)
  line L34 (13.3, 13.5981) -> (10.3, 13.5981)
  line L35 (10.3, 13.5981) -> (8.8, 11)
  line L36 (-3.2, 11) -> (-1.7, 8.4019)
  line L37 (-1.7, 8.4019) -> (1.3, 8.4019)
  line L38 (1.3, 8.4019) -> (2.8, 11)
  line L39 (2.8, 11) -> (1.3, 13.5981)
  line L40 (1.3, 13.5981) -> (-1.7, 13.5981)
  line L41 (-1.7, 13.5981) -> (-3.2, 11)
  line L42 (2.8, 14.5) -> (4.3, 11.9019)
  line L43 (4.3, 11.9019) -> (7.3, 11.9019)
  line L44 (7.3, 11.9019) -> (8.8, 14.5)
  line L45 (8.8, 14.5) -> (7.3, 17.0981)
  line L46 (7.3, 17.0981) -> (4.3, 17.0981)
  line L47 (4.3, 17.0981) -> (2.8, 14.5)
  line L48 (14.8, 14.5) -> (16.3, 11.9019)
  line L49 (16.3, 11.9019) -> (19.3, 11.9019)
  line L50 (19.3, 11.9019) -> (20.8, 14.5)
  line L51 (20.8, 14.5) -> (19.3, 17.0981)
  line L52 (16.3, 17.0981) -> (14.8, 14.5)
  line L53 (19.3, 17.0981) -> (16.3, 17.0981)
  line L54 (26.8, 14.5) -> (28.3, 11.9019)
  line L55 (28.3, 11.9019) -> (31.3, 11.9019)
  line L56 (31.3, 11.9019) -> (32.8, 14.5)
  line L57 (32.8, 14.5) -> (31.3, 17.0981)
  line L58 (28.3, 17.0981) -> (26.8, 14.5)
  line L59 (31.3, 17.0981) -> (28.3, 17.0981)
  line L60 (38.8, 14.5) -> (40.3, 11.9019)
  line L61 (40.3, 11.9019) -> (43.3, 11.9019)
  line L62 (43.3, 11.9019) -> (44.8, 14.5)
  line L63 (44.8, 14.5) -> (43.3, 17.0981)
  line L64 (40.3, 17.0981) -> (38.8, 14.5)
  line L65 (43.3, 17.0981) -> (40.3, 17.0981)
  line L66 (50.8, 14.5) -> (52.3, 11.9019)
  line L67 (52.3, 11.9019) -> (55.3, 11.9019)
  line L68 (55.3, 11.9019) -> (56.8, 14.5)
  line L69 (56.8, 14.5) -> (55.3, 17.0981)
  line L70 (52.3, 17.0981) -> (50.8, 14.5)
  line L71 (55.3, 17.0981) -> (52.3, 17.0981)
  line L72 (-3.2, 18) -> (-1.7, 15.4019)
  line L73 (-1.7, 15.4019) -> (1.3, 15.4019)
  line L74 (1.3, 15.4019) -> (2.8, 18)
  line L75 (2.8, 18) -> (1.3, 20.5981)
  line L76 (1.3, 20.5981) -> (-1.7, 20.5981)
  line L77 (-1.7, 20.5981) -> (-3.2, 18)
  line L78 (2.8, 21.5) -> (4.3, 18.9019)
  line L79 (4.3, 18.9019) -> (7.3, 18.9019)
  line L80 (7.3, 18.9019) -> (8.8, 21.5)
  line L81 (8.8, 21.5) -> (7.3, 24.0981)
  line L82 (4.3, 24.0981) -> (2.8, 21.5)
  line L83 (7.3, 24.0981) -> (4.3, 24.0981)
  line L84 (8.8, 18) -> (10.3, 15.4019)
  line L85 (10.3, 15.4019) -> (13.3, 15.4019)
  line L86 (13.3, 15.4019) -> (14.8, 18)
  line L87 (14.8, 18) -> (13.3, 20.5981)
  line L88 (10.3, 20.5981) -> (8.8, 18)
  line L89 (13.3, 20.5981) -> (10.3, 20.5981)
  line L90 (14.8, 21.5) -> (16.3, 18.9019)
  line L91 (16.3, 18.9019) -> (19.3, 18.9019)
  line L92 (19.3, 18.9019) -> (20.8, 21.5)
  line L93 (20.8, 21.5) -> (19.3, 24.0981)
  line L94 (16.3, 24.0981) -> (14.8, 21.5)
  line L95 (19.3, 24.0981) -> (16.3, 24.0981)
  line L96 (20.8, 18) -> (22.3, 15.4019)
  line L97 (22.3, 15.4019) -> (25.3, 15.4019)
  line L98 (25.3, 15.4019) -> (26.8, 18)
  line L99 (26.8, 18) -> (25.3, 20.5981)
  line L100 (22.3, 20.5981) -> (20.8, 18)
  line L101 (25.3, 20.5981) -> (22.3, 20.5981)
  line L102 (26.8, 21.5) -> (28.3, 18.9019)
  line L103 (28.3, 18.9019) -> (31.3, 18.9019)
  line L104 (31.3, 18.9019) -> (32.8, 21.5)
  line L105 (32.8, 21.5) -> (31.3, 24.0981)
  line L106 (28.3, 24.0981) -> (26.8, 21.5)
  line L107 (31.3, 24.0981) -> (28.3, 24.0981)
  line L108 (32.8, 18) -> (34.3, 15.4019)
  line L109 (34.3, 15.4019) -> (37.3, 15.4019)
  line L110 (37.3, 15.4019) -> (38.8, 18)
  line L111 (38.8, 18) -> (37.3, 20.5981)
  line L112 (34.3, 20.5981) -> (32.8, 18)
  line L113 (37.3, 20.5981) -> (34.3, 20.5981)
  line L114 (38.8, 21.5) -> (40.3, 18.9019)
  line L115 (40.3, 18.9019) -> (43.3, 18.9019)
  line L116 (43.3, 18.9019) -> (44.8, 21.5)
  line L117 (44.8, 21.5) -> (43.3, 24.0981)
  line L118 (40.3, 24.0981) -> (38.8, 21.5)
  line L119 (43.3, 24.0981) -> (40.3, 24.0981)
  line L120 (44.8, 18) -> (46.3, 15.4019)
  line L121 (46.3, 15.4019) -> (49.3, 15.4019)
  line L122 (49.3, 15.4019) -> (50.8, 18)
  line L123 (50.8, 18) -> (49.3, 20.5981)
  line L124 (46.3, 20.5981) -> (44.8, 18)
  line L125 (49.3, 20.5981) -> (46.3, 20.5981)
  line L126 (50.8, 21.5) -> (52.3, 18.9019)
  line L127 (52.3, 18.9019) -> (55.3, 18.9019)
  line L128 (55.3, 18.9019) -> (56.8, 21.5)
  line L129 (56.8, 21.5) -> (55.3, 24.0981)
  line L130 (52.3, 24.0981) -> (50.8, 21.5)
  line L131 (55.3, 24.0981) -> (52.3, 24.0981)
  line L132 (-3.2, 4) -> (-1.7, 1.4019)
  line L133 (-1.7, 1.4019) -> (1.3, 1.4019)
  line L134 (1.3, 1.4019) -> (2.8, 4)
  line L135 (2.8, 4) -> (1.3, 6.5981)
  line L136 (1.3, 6.5981) -> (-1.7, 6.5981)
  line L137 (-1.7, 6.5981) -> (-3.2, 4)
  line L138 (2.8, 7.5) -> (4.3, 4.9019)
  line L139 (4.3, 4.9019) -> (7.3, 4.9019)
  line L140 (7.3, 4.9019) -> (8.8, 7.5)
  line L141 (8.8, 7.5) -> (7.3, 10.0981)
  line L142 (4.3, 10.0981) -> (2.8, 7.5)
  line L143 (7.3, 10.0981) -> (4.3, 10.0981)
  line L144 (8.8, 4) -> (10.3, 1.4019)
  line L145 (10.3, 1.4019) -> (13.3, 1.4019)
  line L146 (13.3, 1.4019) -> (14.8, 4)
  line L147 (14.8, 4) -> (13.3, 6.5981)
  line L148 (10.3, 6.5981) -> (8.8, 4)
  line L149 (13.3, 6.5981) -> (10.3, 6.5981)
  line L150 (14.8, 7.5) -> (16.3, 4.9019)
  line L151 (16.3, 4.9019) -> (19.3, 4.9019)
  line L152 (19.3, 4.9019) -> (20.8, 7.5)
  line L153 (20.8, 7.5) -> (19.3, 10.0981)
  line L154 (16.3, 10.0981) -> (14.8, 7.5)
  line L155 (19.3, 10.0981) -> (16.3, 10.0981)
  line L156 (20.8, 4) -> (22.3, 1.4019)
  line L157 (22.3, 1.4019) -> (25.3, 1.4019)
  line L158 (25.3, 1.4019) -> (26.8, 4)
  line L159 (26.8, 4) -> (25.3, 6.5981)
  line L160 (22.3, 6.5981) -> (20.8, 4)
  line L161 (25.3, 6.5981) -> (22.3, 6.5981)
  line L162 (26.8, 7.5) -> (28.3, 4.9019)
  line L163 (28.3, 4.9019) -> (31.3, 4.9019)
  line L164 (31.3, 4.9019) -> (32.8, 7.5)
  line L165 (32.8, 7.5) -> (31.3, 10.0981)
  line L166 (28.3, 10.0981) -> (26.8, 7.5)
  line L167 (31.3, 10.0981) -> (28.3, 10.0981)
  line L168 (32.8, 4) -> (34.3, 1.4019)
  line L169 (34.3, 1.4019) -> (37.3, 1.4019)
  line L170 (37.3, 1.4019) -> (38.8, 4)
  line L171 (38.8, 4) -> (37.3, 6.5981)
  line L172 (34.3, 6.5981) -> (32.8, 4)
  line L173 (37.3, 6.5981) -> (34.3, 6.5981)
  line L174 (38.8, 7.5) -> (40.3, 4.9019)
  line L175 (40.3, 4.9019) -> (43.3, 4.9019)
  line L176 (43.3, 4.9019) -> (44.8, 7.5)
  line L177 (44.8, 7.5) -> (43.3, 10.0981)
  line L178 (40.3, 10.0981) -> (38.8, 7.5)
  line L179 (43.3, 10.0981) -> (40.3, 10.0981)
  line L180 (44.8, 4) -> (46.3, 1.4019)
  line L181 (46.3, 1.4019) -> (49.3, 1.4019)
  line L182 (49.3, 1.4019) -> (50.8, 4)
  line L183 (50.8, 4) -> (49.3, 6.5981)
  line L184 (46.3, 6.5981) -> (44.8, 4)
  line L185 (49.3, 6.5981) -> (46.3, 6.5981)
  line L186 (50.8, 7.5) -> (52.3, 4.9019)
  line L187 (52.3, 4.9019) -> (55.3, 4.9019)
  line L188 (55.3, 4.9019) -> (56.8, 7.5)
  line L189 (56.8, 7.5) -> (55.3, 10.0981)
  line L190 (52.3, 10.0981) -> (50.8, 7.5)
  line L191 (55.3, 10.0981) -> (52.3, 10.0981)
  line L192 (-3.2, -3) -> (-1.7, -5.5981)
  line L193 (-1.7, -5.5981) -> (1.3, -5.5981)
  line L194 (1.3, -5.5981) -> (2.8, -3)
  line L195 (2.8, -3) -> (1.3, -0.4019)
  line L196 (1.3, -0.4019) -> (-1.7, -0.4019)
  line L197 (-1.7, -0.4019) -> (-3.2, -3)
  line L198 (2.8, 0.5) -> (4.3, -2.0981)
  line L199 (4.3, -2.0981) -> (7.3, -2.0981)
  line L200 (7.3, -2.0981) -> (8.8, 0.5)
  line L201 (8.8, 0.5) -> (7.3, 3.0981)
  line L202 (4.3, 3.0981) -> (2.8, 0.5)
  line L203 (7.3, 3.0981) -> (4.3, 3.0981)
  line L204 (8.8, -3) -> (10.3, -5.5981)
  line L205 (10.3, -5.5981) -> (13.3, -5.5981)
  line L206 (13.3, -5.5981) -> (14.8, -3)
  line L207 (14.8, -3) -> (13.3, -0.4019)
  line L208 (10.3, -0.4019) -> (8.8, -3)
  line L209 (13.3, -0.4019) -> (10.3, -0.4019)
  line L210 (14.8, 0.5) -> (16.3, -2.0981)
  line L211 (16.3, -2.0981) -> (19.3, -2.0981)
  line L212 (19.3, -2.0981) -> (20.8, 0.5)
  line L213 (20.8, 0.5) -> (19.3, 3.0981)
  line L214 (16.3, 3.0981) -> (14.8, 0.5)
  line L215 (19.3, 3.0981) -> (16.3, 3.0981)
  line L216 (20.8, -3) -> (22.3, -5.5981)
  line L217 (22.3, -5.5981) -> (25.3, -5.5981)
  line L218 (25.3, -5.5981) -> (26.8, -3)
  line L219 (26.8, -3) -> (25.3, -0.4019)
  line L220 (22.3, -0.4019) -> (20.8, -3)
  line L221 (25.3, -0.4019) -> (22.3, -0.4019)
  line L222 (26.8, 0.5) -> (28.3, -2.0981)
  line L223 (28.3, -2.0981) -> (31.3, -2.0981)
  line L224 (31.3, -2.0981) -> (32.8, 0.5)
  line L225 (32.8, 0.5) -> (31.3, 3.0981)
  line L226 (28.3, 3.0981) -> (26.8, 0.5)
  line L227 (31.3, 3.0981) -> (28.3, 3.0981)
  line L228 (32.8, -3) -> (34.3, -5.5981)
  line L229 (34.3, -5.5981) -> (37.3, -5.5981)
  line L230 (37.3, -5.5981) -> (38.8, -3)
  line L231 (38.8, -3) -> (37.3, -0.4019)
  line L232 (34.3, -0.4019) -> (32.8, -3)
  line L233 (37.3, -0.4019) -> (34.3, -0.4019)
  line L234 (38.8, 0.5) -> (40.3, -2.0981)
  line L235 (40.3, -2.0981) -> (43.3, -2.0981)
  line L236 (43.3, -2.0981) -> (44.8, 0.5)
  line L237 (44.8, 0.5) -> (43.3, 3.0981)
  line L238 (40.3, 3.0981) -> (38.8, 0.5)
  line L239 (43.3, 3.0981) -> (40.3, 3.0981)
  line L240 (44.8, -3) -> (46.3, -5.5981)
  line L241 (46.3, -5.5981) -> (49.3, -5.5981)
  line L242 (49.3, -5.5981) -> (50.8, -3)
  line L243 (50.8, -3) -> (49.3, -0.4019)
  line L244 (46.3, -0.4019) -> (44.8, -3)
  line L245 (49.3, -0.4019) -> (46.3, -0.4019)
  line L246 (50.8, 0.5) -> (52.3, -2.0981)
  line L247 (52.3, -2.0981) -> (55.3, -2.0981)
  line L248 (55.3, -2.0981) -> (56.8, 0.5)
  line L249 (56.8, 0.5) -> (55.3, 3.0981)
  line L250 (52.3, 3.0981) -> (50.8, 0.5)
  line L251 (55.3, 3.0981) -> (52.3, 3.0981)
  line L252 (30.93, 10) -> (32.93, 10) construction
  line L253 (32.93, 10) -> (32.93, 12) construction
  line L254 (32.93, 12) -> (30.93, 12) construction
  line L255 (30.93, 12) -> (30.93, 10) construction
  line L256 (14.33, 3) -> (12.33, 3) construction
  line L257 (12.33, 3) -> (12.33, 1) construction
  line L258 (12.33, 1) -> (14.33, 1) construction
  line L259 (14.33, 1) -> (14.33, 3) construction
  line L260 (32.93, 12) -> (12.33, 12)
  line L261 (12.33, 12) -> (12.33, 1)
  line L262 (12.33, 1) -> (32.93, 1)
  line L263 (32.93, 1) -> (32.93, 12)
  line L264 (8.8, 11) -> (12.33, 11)
  line L265 (32.8, 11) -> (38.8, 11)
  line L266 (44.8, 11) -> (45.6, 11)
  line L267 (2.8, 11) -> (2, 11)
  point P0 (23.8, 11)
  point P1 (22.3, 15.4019)
  point P2 (22.3, 15.4019)
  point P3 (23.8, 11)
  dimension "d101" = 2
  dimension "d102" = 2
  dimension "d103" = 2
  measures "d101" distance of L0.end L254.end
  measures "d102" distance of L2.end L256.end
  measures "d103" distance of L2.end L258.end
extrude "Extrude14" cut sketch "USB Honeycomb" against normal blind 2 contours L10 L144 L148 L149 L261 | L30 L31 L261 L264 | L0 L1 L163 L164 L165 L166 L167 | L0 L1 L162 L163 L166 | L12 L13 L14 L260 | L33 L34 L35 L260 L261 L264 | L48 L50 L51 L52 L53 L260 | L10 L201 L202 L203 | L54 L56 L57 L58 L59 L260 | L1 L2 L10 L225 L226 L227 | L1 L2 L226 L227 | L11 L134 L135 | L23 L263 L265 | L21 L22 L23 L263 L265 | L18 L263 L265 | L18 L19 L20 L263 L265 | L10 L168 L170 L171 L172 L173 L263 | L168 L172 L263 | L11 L38 L267 | L11 L39 L267 | L10 L237 L238 L239 | L11 L74 L75 | L9 L180 L184 | L8 L78 L79 L80 | L9 L24 L266 | L9 L29 L266 | L8 L84 L85 L86 L87 L88 | L9 L120 L124 | L8 L90 L91 L92 | L8 L114 L115 L116 | L8 L96 L97 L98 L99 L100 | L8 L102 L103 L104 | L8 L108 L109 L110 L111 L112 | L42 L43 L44 L45 L46 L47 | L60 L61 L62 L63 L64 L65 | L138 L139 L140 L141 L142 L143 | L174 L175 L176 L177 L178 L179 bodies 2
sketch "Bottom Cutout" plane through (0, 0, 0) normal (0, 1, 0) x (1, 0, 0)
  line L0 (82.9, -2.1) -> (51.9, -2.1) construction
  line L1 (82.9, -29.5) -> (82.9, -2.1) construction
  line L2 (51.9, -2.1) -> (68.9, -2.1)
  line L3 (68.9, -2.1) -> (68.9, -21.1)
  line L4 (68.9, -21.1) -> (51.9, -21.1)
  line L5 (51.9, -21.1) -> (51.9, -2.1)
  line L6 (82.9, -29.5) -> (64.65, -29.5)
  line L7 (64.65, -29.5) -> (64.65, -10.5)
  line L8 (64.65, -10.5) -> (82.9, -10.5)
  line L9 (82.9, -10.5) -> (82.9, -29.5)
  line L10 (62.65, -31.5) -> (84.9, -31.5) construction
  line L11 (84.9, -31.5) -> (84.9, -8.5) construction
  line L12 (84.9, -8.5) -> (62.65, -8.5)
  line L13 (62.65, -8.5) -> (62.65, -31.5)
  line L14 (78.412, -10.5) -> (78.412, -8.5)
  line L15 (82.9, -12.0985) -> (84.9, -12.0985)
  line L16 (49.858, -0.05) -> (70.858, -0.05)
  line L17 (70.858, -0.05) -> (70.858, -23.05)
  line L18 (70.858, -23.05) -> (49.858, -23.05)
  line L19 (49.858, -23.05) -> (49.858, -0.05)
  line L20 (49.858, -2) -> (70.858, -2)
  circle A0 centre (82.1535, -7.3974) radius 5.9597
  arc A1 (77.8227, -11.5063) -> (82.7771, -13.3173) centre (82.1501, -7.3501) ccw
  arc A2 (77.8227, -11.5063) -> (82.7771, -13.3173) centre (82.1501, -7.3501) ccw
  point P0 (88.9, 0)
  point P1 (60.316, -2)
  point P2 (73.775, -20)
  point P3 (59.6535, -11.7993)
  point P4 (60.358, -11.55)
  point P5 (82.1535, -7.3974)
  point P6 (59.6535, -11.7993)
  dimension "d110" = 17
  dimension "d111" = 19
  dimension "d112" = 18.25
  dimension "d113" = 19
  dimension "d116" = 22.25
  dimension "d117" = 23
  dimension "d124" = 21
  dimension "d125" = 23
  measures "d110" distance of L0.end L2.end
  measures "d111" distance of L0.end L4.end
  measures "d112" distance of L1.start L6.end
  measures "d113" distance of L1.start L8.end
  measures "d116" distance of L11.end L12.end
  measures "d117" distance of L10.end L11.end
  measures "d124" distance of L17.end L18.end
  measures "d125" distance of L16.end L17.end
extrude "Extrude15" cut sketch "Bottom Cutout" along normal blind 2 contours L2 L3 L4 L5 L12 L13 | L3 L4 L7 L8 L12 L13 | L3 L4 L7 L8 bodies 1
extrude "Extrude18" cut sketch "Bottom Cutout" along normal blind 2 contours L2 L3 L4 L5 L12 L13 | L3 L4 L7 L8 L12 L13 | L3 L4 L7 L8 bodies 1
extrude "Extrude21" add sketch "Bottom Cutout" along normal blind 2 contours L8 L9 L12 L14 A0 | L8 L12 L14 A0 | L8 L9 A0 bodies 2 1
extrude "Extrude24" cut sketch "Bottom Honeycomb" along normal blind 2 contours L438 L439 A2 A4 bodies 2
extrude "Extrude25" add sketch "Bottom Honeycomb" along normal blind 2 contours L258 L259 A2 A4 bodies 2
extrude "Extrude26" add sketch "Bottom Honeycomb" along normal blind 2 contours L286 L290 A3 bodies 2
extrude "Extrude27" cut sketch "Bottom Honeycomb" along normal blind 2 contours L352 L356 A0 L560 L565 L568 L569 bodies 2
extrude "Extrude28" add sketch "Bottom Honeycomb" along normal blind 2 contours L352 L356 A0 L560 L565 L568 L569 bodies 2
sketch "Partition" plane through (0, 0, 0) normal (0, 1, 0) x (1, 0, 0)
  line L0 (47.1137, -31.3501) -> (88.9, -31.3501)
  line L1 (88.9, -31.3501) -> (88.9, -33.3501)
  line L2 (88.9, -33.3501) -> (47.1137, -33.3501)
  line L3 (47.1137, -33.3501) -> (47.1137, -31.3501)
  line L4 (47.1137, -33.3501) -> (45.1137, -33.3501)
  line L5 (45.1137, -33.3501) -> (45.1137, 0)
  line L6 (45.1137, 0) -> (47.1137, 0)
  line L7 (47.1137, 0) -> (47.1137, -33.3501)
  point P0 (47.1137, -31.3501)
  dimension "d158" = 2
  dimension "d159" = 2
  measures "d158" distance of P0 L2.end
  measures "d159" distance of L2.end L4.end
extrude "Extrude53" cut sketch "Partition" along normal blind 9 bodies 2
extrude "Extrude54" cut sketch "Partition" along normal blind 9.25 bodies 2
extrude "Extrude55" add sketch "Partition" along normal blind 9.25 bodies 2
extrude "Extrude56" cut sketch "Bottom Cutout" along normal blind 2 contours L2 L3 L4 L5 L12 L13 L17 L18 L19 L20 | L3 L8 L12 L17 | L4 L7 L13 L18 | L3 L4 L7 L8 L17 L18 bodies 2
extrude "Extrude57" add sketch "Bottom Cutout" along normal blind 2 contours L2 L3 L4 L5 L12 L13 L17 L18 L19 L20 | L3 L8 L12 L17 | L4 L7 L13 L18 | L3 L4 L7 L8 L17 L18 bodies 2
extrude "Extrude58" cut sketch "Nut Holes" along normal blind 6 contours L12 L13 L14 L15 L16 L17 bodies 2
extrude "Extrude59" add sketch "USB Honeycomb" against normal blind 2 contours L12 L13 L14 L260 | L33 L34 L35 L260 L261 L264 | L48 L50 L51 L52 L53 L260 | L54 L56 L57 L58 L59 L260 | L21 L22 L23 L263 L265 | L11 L39 L267 | L11 L74 L75 | L8 L78 L79 L80 | L9 L29 L266 | L8 L84 L85 L86 L87 L88 | L9 L120 L124 | L8 L90 L91 L92 | L8 L114 L115 L116 | L8 L96 L97 L98 L99 L100 | L8 L102 L103 L104 | L8 L108 L109 L110 L111 L112 | L42 L43 L44 L45 L46 L47 | L60 L61 L62 L63 L64 L65 bodies 2
extrude "Extrude60" add sketch "USB Honeycomb" against normal blind 2 contours L0 L1 L163 L164 L165 L166 L167 | L1 L2 L10 L225 L226 L227 | L23 L263 L265 | L18 L263 L265 bodies 2
extrude "Extrude61" cut sketch "Fan Mount" along normal blind 2 contours A0 | A1 | A2 | A3 | A4 | A5 A11 | A6 | A7 A8 A9 A10 picked at (10.8366, -5.3897) bodies 2
extrude "Extrude62" add sketch "Fan Mount" along normal blind 2 contours A1 | A2 | A5 A11 | A7 A8 A9 A10 picked at (10.8366, -5.3897) bodies 2
extrude "Extrude63" cut sketch "Bottom Honeycomb" along normal blind 2 contours L322 L326 L327 A7 bodies 2
extrude "Extrude64" add sketch "Bottom Honeycomb" along normal blind 2 contours L322 L326 L327 A7 bodies 2
extrude "Extrude65" add sketch "Bottom Honeycomb" along normal blind 2 contours L334 L338 L339 A8 bodies 2
extrude "Extrude29" [suppressed]
extrude "Extrude30" [suppressed]
extrude "Extrude31" [suppressed]
extrude "Extrude32" [suppressed]
extrude "Extrude33" [suppressed]
extrude "Extrude34" [suppressed]
extrude "Extrude35" [suppressed]
extrude "Extrude36" [suppressed]
extrude "Extrude37" [suppressed]
extrude "Extrude38" [suppressed]
extrude "Extrude39" [suppressed]
extrude "Extrude40" [suppressed]
delete_face "DeleteFace1" [suppressed]
extrude "Extrude43" [suppressed]
extrude "Extrude44" [suppressed]
extrude "Extrude46" [suppressed]
extrude "Extrude47" [suppressed]
extrude "Extrude48" [suppressed]
extrude "Extrude49" [suppressed]
extrude "Extrude50" [suppressed]
extrude "Extrude51" [suppressed]
extrude "Extrude52" [suppressed]
extrude "Extrude45" [suppressed]
